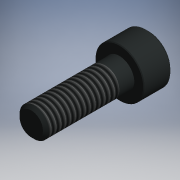
# Autodesk Inventor part: DIN-912 - M6x18(F)
Saved by Autodesk Inventor 2017.3 (Build 213256000, 256)
## iProperties
Part Number: DIN-912 - M6x18(F)
Material: Generic
Catalog Web Link: www.cadenas.de
Description: DIN-912-Cylinder screw
Vendor: FESTO
Document SubType Name: Modeling
Designer: partserver
Manufacturer: FESTO
Mass: 0.896325 g
Surface Area: 7.14969 cm^2
Volume: 0.896325 cm^3
Density: 1 g/cm^3
Appearance: PSOLRGB-46-51-51
Category: PARTsolutions
Company: FESTO
Title: DIN-912 - M6x18(F)
Author: Cadenas PARTsolutions
Comments: Cylinder screw
PSOL_IDENT_0: {$CADENAS_DATA\23d-libs\festo\zyl_zubeh\d912\din_912.prj},179 {VTYP=3D},{NB=DIN-912 - M6x18(F)},{LIN
PSOL_IDENT_1: A=DIN-912 - M6x18(F)},{NN=DIN-912},{DATE=01.07.2020 05:33:41},{GEOMDATE=01.07.2020 05:33:34},{VERSIO
PSOL_IDENT_2: N=},{LINEID=1230},{WBVAR=},{WBNUMERIC=}  {NB=DIN-912 - M6x18(F)},{LINA=DIN-912 - M6x18(F)},{KT=X},{I
PSOL_IDENT_3: DNR=},{GEW=M6},{DG=6.000},{P=1.000},{L=18.000},{B=18.000},{FORM=1},{GKD=4.773},{DK=10.000},{DADIN=6.
PSOL_IDENT_4: 800},{DS=6.000},{E=5.720},{LF=0.680},{K=6.000},{R=0.250},{S=5.000},{T=3.000},{V=0.600},{DW=9.380},{W=
PSOL_IDENT_5: 2.300},{NENN=M6x18},{DA=6.1},{BL=15}
NB: DIN-912 - M6x18(F)
NN: DIN-912
NT: Cylinder screw
NBSYN: DIN-912 - $NENN.(F)
LINA: DIN-912 - M6x18(F)
CATALOG: Festo
ROWDESC: M6x18
GEW: M6
DG: 6
P: 1
L: 18
B: 18
FORM: 1
GKD: 4.773
DK: 10
DADIN: 6.8
DS: 6
E: 5.72
LF: 0.68
K: 6
R: 0.25
S: 5
T: 3
V: 0.6
DW: 9.38
W: 2.3
SUPPLIER: FESTO
ARTICLENO: DIN-912 - M6x18(F)
BOMINFO: DIN-912 - M6x18(F)
CREATOR: CADENAS GmbH
Autodesk Inventor part; units mm, degrees
sketch "Sketch_1" plane through (0, 0, 0) normal (0, 0, 1) x (1, 0, 0)
  line L0 (0, -18) -> (0, 6)
  line L1 (0, 1.5566) -> (2.5, 3)
  line L2 (2.5, 3) -> (2.5, 5.6132)
  line L3 (2.5, 5.6132) -> (2.8868, 6)
  line L4 (2.8868, 6) -> (4.4, 6)
  line L5 (4.4, 6) -> (5, 5.4)
  line L6 (5, 5.4) -> (5, 0.15)
  line L7 (5, 0.15) -> (4.85, 0)
  line L8 (4.85, 0) -> (3.05, 0)
  line L9 (3.05, 0) -> (3, -0.68)
  line L10 (3, -0.68) -> (3, -17.3865)
  line L11 (3, -17.3865) -> (2.3865, -18)
  line L12 (2.3865, -18) -> (0, -18)
  line L13 (0, -18) -> (0, 1.5566)
  constraints: 28 end point
revolve "Revolution1" add sketch "Sketch_1" angle 360 about axis through (0, -18, 0) along (0, -1, 0)
thread "Thread1" size "M6x1" class "6g" standard "ISO Metric profile" length 14.3865
sketch "Sketch_2" plane through (0, 6, 0) normal (0, 1, 0) x (1, 0, 0)
  line L0 (-2.5, -1.4434) -> (0, -2.8868)
  line L1 (0, -2.8868) -> (2.5, -1.4434)
  line L2 (2.5, -1.4434) -> (2.5, 1.4434)
  line L3 (2.5, 1.4434) -> (0, 2.8868)
  line L4 (0, 2.8868) -> (-2.5, 1.4434)
  line L5 (-2.5, 1.4434) -> (-2.5, -1.4434)
  constraints: 12 end point
extrude "Extrusion1" cut sketch "Sketch_2" against normal blind 3
ref_plane "ANBAU_XY" through (0, 0, 0) normal (0, 1, 0) x (1, 0, 0)
ref_plane "ANBAU_YZ" through (0, 0, 0) normal (1, 0, 0) x (0, 0, -1)
ref_plane "ANBAU_ZX" through (0, 0, 0) normal (0, 0, -1) x (0, 1, 0)
ref_plane "Schraube_XY" through (0, 0, 0) normal (0, 1, 0) x (1, 0, 0)
ref_plane "Schraube_YZ" through (0, 0, 0) normal (1, 0, 0) x (0, 0, -1)
ref_plane "Schraube_ZX" through (0, 0, 0) normal (0, 0, -1) x (0, 1, 0)
ref_plane "insert_XY" through (0, 0, 0) normal (0, 1, 0) x (1, 0, 0)
ref_plane "insert_YZ" through (0, 0, 0) normal (1, 0, 0) x (0, 0, -1)
ref_plane "insert_ZX" through (0, 0, 0) normal (0, 0, -1) x (0, 1, 0)
ref_plane "schrauben_punkt_XY" through (0, -18, 0) normal (0, 1, 0) x (1, 0, 0)
ref_plane "schrauben_punkt_YZ" through (0, -18, 0) normal (1, 0, 0) x (0, 0, -1)
ref_plane "schrauben_punkt_ZX" through (0, -18, 0) normal (0, 0, -1) x (0, 1, 0)
body "Solid1"
